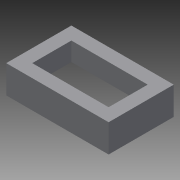
# Autodesk Inventor part: embudo0.2
Saved by Autodesk Inventor 2015 SP1 (Build 190203100, 203)
## iProperties
Created: 2015-07-20
Part Number: embudo0.2
Material: Generic
Document SubType Name: Modeling
Designer: pc
Density: 1 g/cm^3
Appearance: Default
Author: pc
Autodesk Inventor part; units mm, degrees
ref_plane "Work Plane1" through (0, 0, 80) normal (0, 0, 1) x (1, 0, 0)
ref_plane "YZ Plane" through (0, 0, 0) normal (1, 0, 0) x (0, 1, 0)
ref_plane "XZ Plane" through (0, 0, 0) normal (0, 1, 0) x (-1, 0, 0)
sketch "Sketch4" plane through (0, 0, 0) normal (0, 0, 1) x (1, 0, 0)
  line L0 (-27.5, 17.5) -> (27.5, 17.5)
  line L1 (27.5, 17.5) -> (27.5, -17.5)
  line L2 (27.5, -17.5) -> (-27.5, -17.5)
  line L3 (-27.5, -17.5) -> (-27.5, 17.5)
  line L4 (0, 0) -> (0, -2.5)
  line L5 (0, 0) -> (1.7044, 0)
  dimension "d52" = 55
  dimension "d53" = 35
  constraints: 12 end point, 2 horizontal, 2 parallel, 2 symmetric about line, 1 perpendicular
  measures "d52" distance of L0.start L0.end
  measures "d53" distance of L0.end L1.end
extrude "Extrusion3" add sketch "Sketch4" along normal blind 15
sketch "Sketch1" plane through (0, 0, 0) normal (0, 0, -1) x (-1, 0, 0)
  line L0 (-25.5, 15.5) -> (25.5, 15.5)
  line L1 (25.5, 15.5) -> (25.5, -15.5)
  line L2 (25.5, -15.5) -> (-25.5, -15.5)
  line L3 (-25.5, -15.5) -> (-25.5, 15.5)
  line L4 (27.5, 17.5) -> (-27.5, 17.5) projected
  line L5 (-27.5, 17.5) -> (-27.5, -17.5) projected
  line L6 (-27.5, -17.5) -> (27.5, -17.5) projected
  line L7 (27.5, -17.5) -> (27.5, 17.5) projected
  line L8 (0, 0) -> (0, -2)
  line L9 (0, 0) -> (2, 0)
  dimension "d0" = 51
  dimension "d1" = 31
  constraints: 12 end point, 2 horizontal, 2 parallel, 2 symmetric about line, 1 perpendicular, 1 vertical
  measures "d0" distance of L0.start L0.end
  measures "d1" distance of L2.end L0.start
extrude "Extrusion4" cut sketch "Sketch1" against normal blind 10 contours L0 L1 L2 L3
sketch "Sketch5" plane through (0, 0, 10) normal (0, 0, -1) x (-1, 0, 0)
  line L0 (-25.5, 15.5) -> (25.5, 15.5) projected
  line L1 (-25.5, -15.5) -> (-25.5, 15.5) projected
  line L2 (25.5, -15.5) -> (-25.5, -15.5) projected
  line L3 (25.5, 15.5) -> (25.5, -15.5) projected
  line L4 (0, 0) -> (2, 0)
  line L5 (0, 0) -> (0, -2)
  line L6 (-20.5, 10.5) -> (20.5, 10.5)
  line L7 (20.5, 10.5) -> (20.5, -10.5)
  line L8 (20.5, -10.5) -> (-20.5, -10.5)
  line L9 (-20.5, -10.5) -> (-20.5, 10.5)
  dimension "d58" = 2
  dimension "d59" = 2
  dimension "d60" = 41
  dimension "d61" = 21
  constraints: 12 end point, 2 horizontal, 2 parallel, 2 symmetric about line, 1 perpendicular, 1 vertical
  measures "d58" distance of L4.start L4.end
  measures "d59" distance of L4.start L5.end
  measures "d60" distance of L6.start L6.end
  measures "d61" distance of L8.end L6.start
extrude "Extrusion5" cut sketch "Sketch5" against normal blind 5 contours L6 L7 L8 L9
sketch "Sketch2" plane through (0, 0, 80) normal (0, 0, 1) x (1, 0, 0)
  circle A0 centre (0, 0) radius 55
  dimension "d6" = 110
  constraints: 1 centre point, 1 coincident
  measures "d6" diameter of A0
sketch "Sketch3" plane through (0, 0, 80) normal (0, 0, 1) x (1, 0, 0)
  circle A0 centre (0, 0) radius 52
  dimension "d30" = 104
  constraints: 1 centre point, 1 coincident
  measures "d30" diameter of A0
body "Solid1"
body "Solid2"
